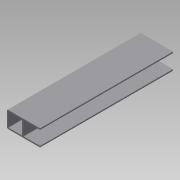
# Autodesk Inventor part: 9725
Saved by Autodesk Inventor 2013 (Build 170138000, 138)
## iProperties
Created: 2014-04-23
Part Number: 9725
Material: Generic
Document SubType Name: Modeling
Density: 1 g/cm^3
Vendor: 80/20 Inc.
Engineer: Ross Bowman
Designer: Ross Bowman
Catalog Web Link: 8020.net
Company: 80/20 Inc.
Author: Ross Bowman
Keywords: 80/20 , 8020 , T-Slot , Extrusion
Material: 6105-T5 Aluminum
Autodesk Inventor part; units mm, degrees
ref_plane "YZ Plane" through (0, 0, 0) normal (1, 0, 0) x (0, 1, 0)
ref_plane "XZ Plane" through (0, 0, 0) normal (0, 1, 0) x (-1, 0, 0)
ref_plane "XY Plane" through (0, 0, 0) normal (0, 0, 1) x (1, 0, 0)
sketch "Sketch1" plane through (0, 0, 0) normal (0, 0, 1) x (1, 0, 0)
  arc A0 (14.2748, -15.875) -> (15.875, -14.2748) centre (14.2748, -14.2748) ccw
  line L0 (15.875, -14.2748) -> (15.875, 14.2748)
  line L1 (14.2748, 15.875) -> (-14.2748, 15.875)
  arc A1 (-14.2748, 15.875) -> (-15.875, 14.2748) centre (-14.2748, 14.2748) ccw
  line L2 (-15.875, 14.2748) -> (-15.875, -14.2748)
  arc A2 (-15.875, -14.2748) -> (-14.2748, -15.875) centre (-14.2748, -14.2748) ccw
  line L3 (-14.2748, -15.875) -> (14.2748, -15.875)
  arc A3 (15.875, 14.2748) -> (14.2748, 15.875) centre (14.2748, 14.2748) ccw
  line L4 (-15.875, -19.05) -> (56.769, -19.05)
  line L5 (56.769, -19.05) -> (57.15, -18.669)
  line L6 (57.15, -18.669) -> (57.15, -16.256)
  line L7 (57.15, -16.256) -> (56.769, -15.875)
  line L8 (56.769, -15.875) -> (20.6502, -15.875)
  arc A4 (19.05, -14.2748) -> (20.6502, -15.875) centre (20.6502, -14.2748) ccw
  line L9 (19.05, -14.2748) -> (19.05, 14.2748)
  arc A5 (20.6502, 15.875) -> (19.05, 14.2748) centre (20.6502, 14.2748) ccw
  line L10 (20.6502, 15.875) -> (56.769, 15.875)
  line L11 (56.769, 15.875) -> (57.15, 16.256)
  line L12 (57.15, 16.256) -> (57.15, 18.669)
  line L13 (57.15, 18.669) -> (56.769, 19.05)
  line L14 (56.769, 19.05) -> (-15.875, 19.05)
  arc A6 (-15.875, 19.05) -> (-19.05, 15.875) centre (-15.875, 15.875) ccw
  line L15 (-19.05, 15.875) -> (-19.05, -15.875)
  arc A7 (-19.05, -15.875) -> (-15.875, -19.05) centre (-15.875, -15.875) ccw
  point P0 (0, 0)
  constraints: 32 end point, 16 point on circle, 8 centre point
extrude "Extrusion1" add sketch "Sketch1" against normal blind 304.8
body "Solid1"
